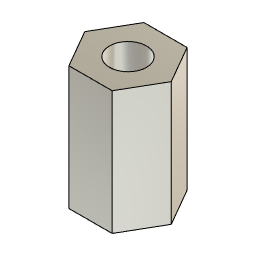
10mmスペーサー (Autodesk Fusion 360 design; units mm, degrees)
Autodesk Fusion 360 part; units mm, degrees
sketch "スケッチ1" plane through (0, 0, 0) normal (0, 0, 1) x (1, 0, 0)
  line L0 (3.5, 0) -> (1.75, 3.0311)
  line L1 (1.75, 3.0311) -> (-1.75, 3.0311)
  line L2 (-1.75, 3.0311) -> (-3.5, 0)
  line L3 (-3.5, 0) -> (-1.75, -3.0311)
  line L4 (-1.75, -3.0311) -> (1.75, -3.0311)
  line L5 (1.75, -3.0311) -> (3.5, 0)
  circle A0 centre (0, 0) radius 1.5
  dimension "d1" = 3
  constraint coincident A0.centre origin
  measures "d1" diameter of A0
extrude "押し出し1" add sketch "スケッチ1" along normal blind 10
